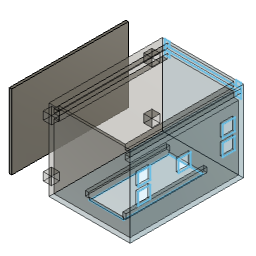
box_ver4 v3 (Autodesk Fusion 360 design; units mm, degrees)
Autodesk Fusion 360 part; units mm, degrees
sketch "Sketch1" plane through (0, 0, 0) normal (0, 1, 0) x (1, 0, 0)
  line L0 (0, 0) -> (100, 0)
  line L1 (100, 0) -> (100, -100)
  line L2 (100, -100) -> (0, -100)
  line L3 (0, -100) -> (0, 0)
  constraint horizontal L0
  constraint vertical L1
  constraint horizontal L2
  constraint vertical L3
  constraint coincident L0.start L3.end
extrude "Extrude1" add sketch "Sketch1" along normal blind 140 makes body 1
sketch "Sketch2" plane through (0, 0, 0) normal (0, 0, -1) x (1, 0, 0)
  line L0 (100, 0) -> (0, 0)
  line L1 (0, 0) -> (0, -140)
  line L2 (0, -140) -> (100, -140)
  line L3 (100, -140) -> (100, 0)
  line L4 (71, -118.8211) -> (29, -118.8211)
  line L5 (29, -118.8211) -> (29, -21.0702)
  line L6 (29, -21.0702) -> (71, -21.0702)
  line L7 (71, -21.0702) -> (71, -118.8211)
  constraint horizontal L4
  constraint vertical L5
  constraint horizontal L6
  constraint vertical L7
shell "Shell1" thickness 3 removed faces 1 at (66.6667, 46.6667, 100) on bodies 1
extrude "Extrude2" cut sketch "Sketch2" against normal blind 3 contours L4 L5 L6 L7 bodies 1
other "Base Mesh Feature1"
other "Base Mesh Feature2"
mesh_step "MeshCombine1"
other "Modify1"
other "Modify2"
sketch "Sketch4" plane through (0, 0, 3) normal (0, 0, 1) x (1, 0, 0)
  line L0 (71, 120) -> (75, 120)
  line L1 (75, 120) -> (75, 20)
  line L2 (75, 20) -> (71, 20)
  line L3 (71, 20) -> (71, 120)
  line L4 (25, 120) -> (29, 120)
  line L5 (29, 120) -> (29, 20)
  line L6 (29, 20) -> (25, 20)
  line L7 (25, 20) -> (25, 120)
  constraint horizontal L0
  constraint vertical L1
  constraint horizontal L2
  constraint vertical L3
  constraint horizontal L4
  constraint vertical L5
  constraint horizontal L6
  constraint vertical L7
extrude "Extrude3" add sketch "Sketch4" along normal blind 6 bodies 1
sketch "Sketch5" plane through (100, 0, 0) normal (1, 0, 0) x (0, 1, 0)
  line L0 (0, 100) -> (0, 0)
  line L1 (0, 0) -> (140, 0)
  line L2 (140, 0) -> (140, 100)
  line L3 (140, 100) -> (0, 100)
  line L4 (10, 50) -> (25, 50)
  line L5 (25, 50) -> (25, 35)
  line L6 (25, 35) -> (10, 35)
  line L7 (10, 35) -> (10, 50)
  line L8 (10.1502, 70.2199) -> (25.1171, 70.2199)
  line L9 (25.1171, 70.2199) -> (25.1171, 55.2199)
  line L10 (25.1171, 55.2199) -> (10.1502, 55.2199)
  line L11 (10.1502, 55.2199) -> (10.1502, 70.2199)
  line L12 (60, 60) -> (75, 60)
  line L13 (75, 60) -> (75, 45)
  line L14 (75, 45) -> (60, 45)
  line L15 (60, 45) -> (60, 60)
  line L16 (114.4945, 69.8554) -> (129.4945, 69.8554)
  line L17 (129.4945, 69.8554) -> (129.4945, 54.8554)
  line L18 (129.4945, 54.8554) -> (114.4945, 54.8554)
  line L19 (114.4945, 54.8554) -> (114.4945, 69.8554)
  line L20 (114.4945, 49.8554) -> (129.4945, 49.8554)
  line L21 (129.4945, 49.8554) -> (129.4945, 34.8554)
  line L22 (129.4945, 34.8554) -> (114.4945, 34.8554)
  line L23 (114.4945, 34.8554) -> (114.4945, 49.8554)
  constraint horizontal L4
  constraint vertical L5
  constraint horizontal L6
  constraint vertical L7
  constraint horizontal L8
  constraint vertical L9
  constraint horizontal L10
  constraint vertical L11
  constraint horizontal L12
  constraint vertical L13
  constraint horizontal L14
  constraint vertical L15
  constraint horizontal L16
  constraint vertical L17
  constraint horizontal L18
  constraint vertical L19
  constraint horizontal L20
  constraint vertical L21
  constraint horizontal L22
  constraint vertical L23
extrude "Extrude4" cut sketch "Sketch5" against normal blind 3 contours L4 L5 L6 L7 | L8 L9 L10 L11 | L12 L13 L14 L15 | L16 L17 L18 L19 | L20 L21 L22 L23 bodies 1
sketch "Sketch6" plane through (0, 140, 0) normal (0, 1, 0) x (-1, 0, 0)
  line L0 (0, 100) -> (-100, 100)
  line L1 (-100, 100) -> (-100, 0)
  line L2 (-100, 0) -> (0, 0)
  line L3 (0, 0) -> (0, 100)
  line L4 (-97, 94) -> (-3, 94)
  line L5 (-3, 94) -> (-3, 89)
  line L6 (-3, 89) -> (-97, 89)
  line L7 (-97, 89) -> (-97, 94)
  constraint horizontal L4
  constraint vertical L5
  constraint horizontal L6
  constraint vertical L7
extrude "Extrude5" cut sketch "Sketch6" against normal up to surface (140 mm away) contours L4 L5 L6 L7 bodies 1
extrude "Extrude6" add sketch "Sketch6" against normal up to surface (140 mm away) separate body contours L4 L5 L6 L7 makes body 2
sketch "Sketch7" plane through (50, 140, 50) normal (0, 1, 0) x (-1, 0, 0)
  line L0 (-47, 50) -> (-41, 50)
  line L1 (-41, 50) -> (-41, 44)
  line L2 (-41, 44) -> (-47, 44)
  line L3 (-47, 44) -> (-47, 50)
  line L4 (-47, 39) -> (-41, 39)
  line L5 (-41, 39) -> (-41, 33)
  line L6 (-41, 33) -> (-47, 33)
  line L7 (-47, 33) -> (-47, 39)
  line L8 (47, 44) -> (41, 44)
  line L9 (41, 44) -> (41, 50)
  line L10 (41, 50) -> (47, 50)
  line L11 (47, 50) -> (47, 44)
  line L12 (47, 39) -> (41, 39)
  line L13 (41, 39) -> (41, 33)
  line L14 (41, 33) -> (47, 33)
  line L15 (47, 33) -> (47, 39)
  constraint horizontal L0
  constraint vertical L1
  constraint horizontal L2
  constraint vertical L3
  constraint horizontal L4
  constraint vertical L5
  constraint horizontal L6
  constraint vertical L7
  constraint horizontal L8
  constraint vertical L9
  constraint horizontal L10
  constraint vertical L11
  constraint horizontal L12
  constraint vertical L13
  constraint horizontal L14
  constraint vertical L15
extrude "Extrude7" add sketch "Sketch7" against normal up to surface (140 mm away) bodies 1 2
extrude "Extrude8" cut sketch "Sketch6" against normal blind 140 contours L4 L5 L6 L7 bodies 1
sketch "Sketch8" plane through (0, 140, 0) normal (0, 1, 0) x (-1, 0, 0)
  line L0 (-96, 93) -> (-4, 93)
  line L1 (-4, 93) -> (-4, 90)
  line L2 (-4, 90) -> (-96, 90)
  line L3 (-96, 90) -> (-96, 93)
  constraint horizontal L0
  constraint vertical L1
  constraint horizontal L2
  constraint vertical L3
extrude "Extrude9" add sketch "Sketch8" along normal blind 144 separate body makes body 3
move_body "Move1" bodies 3 to x (1, 0, 0) y (0, 1, 0) z (0, 0, 1) at (-100, -140, -90)
sketch "Sketch9" plane through (0, 0, 0) normal (-1, 0, 0) x (0, -1, 0)
  line L0 (0, 0) -> (0, 100)
  line L1 (0, 100) -> (-140, 100)
  line L2 (-140, 100) -> (-140, 0)
  line L3 (-140, 0) -> (0, 0)
  line L4 (-137, 85) -> (-127, 85)
  line L5 (-127, 85) -> (-127, 75)
  line L6 (-127, 75) -> (-137, 75)
  line L7 (-137, 75) -> (-137, 85)
  line L8 (-127, 10) -> (-137, 10)
  line L9 (-137, 10) -> (-137, 20)
  line L10 (-137, 20) -> (-127, 20)
  line L11 (-127, 20) -> (-127, 10)
  line L12 (-3, 20) -> (-13, 20)
  line L13 (-13, 20) -> (-13, 10)
  line L14 (-13, 10) -> (-3, 10)
  line L15 (-3, 10) -> (-3, 20)
  line L16 (-3, 85) -> (-13, 85)
  line L17 (-13, 85) -> (-13, 75)
  line L18 (-13, 75) -> (-3, 75)
  line L19 (-3, 75) -> (-3, 85)
  constraint horizontal L4
  constraint vertical L5
  constraint horizontal L6
  constraint vertical L7
  constraint horizontal L8
  constraint vertical L9
  constraint horizontal L10
  constraint vertical L11
  constraint horizontal L12
  constraint vertical L13
  constraint horizontal L14
  constraint vertical L15
  constraint horizontal L16
  constraint vertical L17
  constraint horizontal L18
  constraint vertical L19
extrude "Extrude10" add sketch "Sketch9" along normal blind 10 contours L4 L5 L6 L7 | L8 L9 L10 L11 | L12 L13 L14 L15 | L16 L17 L18 L19 bodies 1
move_body "Move2" bodies 3 to x (1, 0, 0) y (0, 1, 0) z (0, 0, 1) at (-10, 0, 0)
extrude "Extrude11" add sketch "Sketch6" against normal blind 140 contours L4 L5 L6 L7 bodies 1
extrude "Extrude12" cut sketch "Sketch6" against normal up to surface (137 mm away) contours L4 L5 L6 L7 bodies 1
move_body "Move3" bodies 3 to x (0, 0, 1) y (0, 1, 0) z (-1, 0, 0) at (-46, 0, 106)
